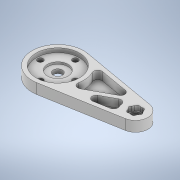
# Autodesk Inventor part: Ankle_side_pitch_frame
Saved by Autodesk Inventor 2020.4 (Build 244396000, 396)
## iProperties
Created: 2021-10-01
Part Number: Ankle_side_pitch_frame
Material: アルミニウム 2014-T4
Document SubType Name: Modeling
Designer: Masato Kubotera
Density: 2.8 g/cm^3
Appearance: 滑らか - 淡い灰色
Description: A2017 T5
Author: Masato Kubotera
Autodesk Inventor part; units mm, degrees
ref_plane "YZ Plane" through (0, 0, 0) normal (1, 0, 0) x (0, 1, 0)
ref_plane "XZ Plane" through (0, 0, 0) normal (0, 1, 0) x (-1, 0, 0)
ref_plane "XY Plane" through (0, 0, 0) normal (0, 0, 1) x (1, 0, 0)
sketch "スケッチ1" plane through (0, 0, 0) normal (0, 0, 1) x (1, 0, 0)
  circle A0 centre (0, 0) radius 10.5 construction
  circle A1 centre (0, 0) radius 5 construction
  circle A2 centre (0, 0) radius 5.01
  circle A3 centre (0, 0) radius 10.51
  arc A4 (2.1531, 12.3132) -> (2.1531, -12.3132) centre (0, 0) ccw
  circle A5 centre (37.7359, 0) radius 2.25
  arc A6 (38.7694, -5.9103) -> (38.7694, 5.9103) centre (37.7359, 0) ccw
  circle A7 centre (8.5, 0) radius 1.35
  circle A8 centre (0, 8.5) radius 1.35
  circle A9 centre (-8.5, 0) radius 1.35
  circle A10 centre (0, -8.5) radius 1.35
  line L0 (2.1531, 12.3132) -> (38.7694, 5.9103)
  line L1 (2.1531, -12.3132) -> (38.7694, -5.9103)
  line L2 (8.4896, 9.1748) -> (32.4358, 4.9875)
  line L3 (34.0196, -4.7105) -> (11.5743, -8.6354)
  arc A11 (2.1531, -12.3132) -> (-4.7001, 11.5827) centre (0, 0) ccw construction
  arc A12 (38.7694, 5.9103) -> (38.7694, -5.9103) centre (37.7359, 0) ccw construction
  line L4 (34.0196, 4.7105) -> (8.4896, -9.1748) construction
  line L5 (32.4358, 4.9875) -> (10.3333, -7.0337)
  line L6 (32.3635, 2.6714) -> (11.5743, -8.6354)
  line L7 (32.4358, 4.9875) -> (34.0196, 4.7105) construction
  line L8 (11.5743, -8.6354) -> (8.4896, -9.1748) construction
  arc A13 (32.3635, 2.6714) -> (34.0196, -4.7105) centre (37.7359, 0) ccw
  arc A14 (10.3333, -7.0337) -> (8.4896, 9.1748) centre (0, 0) ccw
  line L9 (40.9229, 0) -> (40.3979, -0.9093) construction
  line L10 (39.3294, -2.76) -> (38.2794, -2.76) construction
  line L11 (36.1424, -2.76) -> (35.6174, -1.8507) construction
  line L12 (34.549, 0) -> (35.074, 0.9093) construction
  line L13 (36.1424, 2.76) -> (37.1924, 2.76) construction
  line L14 (39.3294, 2.76) -> (39.8544, 1.8507)
  arc A15 (40.3979, -0.9093) -> (40.3979, 0.9093) centre (39.8729, 0) ccw
  arc A16 (39.8544, 1.8507) -> (38.2794, 2.76) centre (38.8044, 1.8507) ccw
  arc A17 (37.1924, 2.76) -> (35.6174, 1.8507) centre (36.6674, 1.8507) ccw
  arc A18 (35.074, 0.9093) -> (35.074, -0.9093) centre (35.599, 0) ccw
  arc A19 (35.6174, -1.8507) -> (37.1924, -2.76) centre (36.6674, -1.8507) ccw
  arc A20 (38.2794, -2.76) -> (39.8544, -1.8507) centre (38.8044, -1.8507) ccw
  line L15 (40.3979, -0.9093) -> (39.8544, -1.8507)
  line L16 (39.8544, -1.8507) -> (39.3294, -2.76) construction
  line L17 (38.2794, -2.76) -> (37.1924, -2.76)
  line L18 (37.1924, -2.76) -> (36.1424, -2.76) construction
  line L19 (35.6174, -1.8507) -> (35.074, -0.9093)
  line L20 (35.074, -0.9093) -> (34.549, 0) construction
  line L21 (35.6174, 1.8507) -> (36.1424, 2.76) construction
  line L22 (35.074, 0.9093) -> (35.6174, 1.8507)
  line L23 (37.1924, 2.76) -> (38.2794, 2.76)
  line L24 (38.2794, 2.76) -> (39.3294, 2.76) construction
  line L25 (39.8544, 1.8507) -> (40.3979, 0.9093)
  line L26 (40.3979, 0.9093) -> (40.9229, 0) construction
  circle A21 centre (37.7359, 0) radius 1.55
  circle A22 centre (0, 0) radius 2.25
  line L27 (0, 0) -> (27.1359, -16.96) construction
  line L28 (37.7359, 0) -> (27.1359, -16.96) construction
  line L29 (0, 0) -> (37.7359, 0) construction
  point P0 (39.3294, 2.76)
  dimension "d0" = 21
  dimension "d1" = 10
  dimension "d2" = 0.01
  dimension "d3" = 0.01
  dimension "d4" = 25
  dimension "d7" = 4.5
  dimension "d8" = 6
  dimension "d9" = 2.7
  dimension "d10" = 8.5
  dimension "d13" = 360
  dimension "d15" = 2
  dimension "d16" = 2
  dimension "d17" = 1
  dimension "d18" = 1
  dimension "d20" = 1.05
  dimension "d23" = 360
  dimension "d25" = 5.52
  dimension "d30" = 3.1
  dimension "d33" = 4.5
  dimension "d41" = 20
  dimension "d42" = 32
  constraints: 60 end point, 32 point on circle, 23 centre point, 14 coincident, 6 parallel, 4 tangent, 3 collinear, 2 point on line, 1 horizontal, 1 perpendicular, 53 other
  measures "d0" diameter of A0
  measures "d1" diameter of A1
  measures "d2" radial gap between concentric circles of A3 A0
  measures "d3" radial gap between concentric circles of A2 A1
  measures "d4" diameter of A4
  measures "d7" diameter of A5
  measures "d8" radius of A6
  measures "d9" diameter of A7
  measures "d10" distance of point (0, 0) A7.centre
  measures "d15" distance between parallel lines of L0 L2
  measures "d16" distance between parallel lines of L1 L3
  measures "d17" distance between parallel lines of L4 L6
  measures "d18" distance between parallel lines of L5 L4
  measures "d20" radius of A15
  measures "d25" distance between parallel lines of L23 L17
  measures "d30" diameter of A21
  measures "d33" diameter of A22
  measures "d41" distance of L28.start L27.end
  measures "d42" distance of L27.start L27.end
extrude "押し出し1" add sketch "スケッチ1" along normal blind 5 contours L0 A6 L1 A4
extrude "押し出し2" add sketch "スケッチ1" along normal blind 2.8 contours L14 L25 A15 L15 A20 L17 A19 L19 A18 L22 A17 L23 A16
extrude "押し出し3" add sketch "スケッチ1" along normal blind 2 contours A5
extrude "押し出し4" add sketch "スケッチ1" along normal blind 3 contours A3
extrude "押し出し5" add sketch "スケッチ1" along normal blind 2 contours A2
extrude "押し出し6" add sketch "スケッチ1" along normal blind 1 contours L2 L5 A14 | L3 L6 A13
fillet "フィレット1" radius 2 6 edges at (8.4896, 9.1748, 3) (10.3333, -7.0337, 3) (11.5743, -8.6354, 3) (32.4358, 4.9875, 3) (32.3635, 2.6714, 3) (34.0196, -4.7105, 3)
equation "\"d3\" = d2"
equation "\"d18\" = d17"
